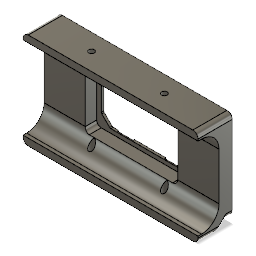
mains_plug_panel-parametric (Autodesk Fusion 360 design; units mm, degrees)
Autodesk Fusion 360 part; units mm, degrees
sketch "Sketch1" plane through (0, 0, 0) normal (1, 0, 0) x (0, 0, -1)
  line L0 (0, 0) -> (0, 51)
  line L1 (0, 51) -> (-20, 51)
  line L2 (-20, 51) -> (-20, 47)
  line L3 (-20, 47) -> (-18, 47)
  line L4 (-18, 47) -> (-8, 47) construction
  line L5 (-8, 47) -> (-8, 37) construction
  arc A0 (-8, 37) -> (-18, 47) centre (-18, 37) ccw
  line L6 (-8, 37) -> (-8, 10)
  line L7 (0, 0) -> (-7, 0)
  line L8 (-7, 0) -> (-11, 0) construction
  line L9 (-11, 0) -> (-11, -4) construction
  line L10 (-7, 0) -> (-11, -4)
  line L11 (-11, -4) -> (-20, -4)
  line L12 (-20, -4) -> (-20, 0)
  line L13 (-20, 0) -> (-18, 0)
  line L14 (-18, 0) -> (-8, 0) construction
  line L15 (-8, 0) -> (-8, 10) construction
  arc A1 (-18, 0) -> (-8, 10) centre (-18, 10) ccw
  line L16 (-8, 10) -> (0, 10) construction
  dimension "d1" = 51
  dimension "d2" = 20
  dimension "d3" = 4
  dimension "d5" = 2
  dimension "d6" = 10
  dimension "d7" = 10
  dimension "d8" = 27
  dimension "d12" = 7
  dimension "d13" = 4
  dimension "d14" = 4
  dimension "d15" = 9
  dimension "d16" = 4
  dimension "d17" = 2
  dimension "d18" = 10
  dimension "d19" = 10
  measures "d1" distance of L0.start
  measures "d2" distance of L0.start
  measures "d5" distance of L0.start
  measures "d12" distance of L0.start
  measures "d16" distance of L0.start
  measures "d17" distance of L0.start
extrude "Extrude1" add sketch "Sketch1" along normal blind 100
sketch "Sketch3" plane through (0, 0, 20) normal (0, 0, 1) x (1, 0, 0)
  line L0 (0, 51) -> (0, 47)
  line L1 (0, 47) -> (100, 47)
  line L2 (100, 47) -> (100, 51)
  line L3 (100, 51) -> (0, 51)
  line L4 (0, -4) -> (100, -4)
  line L5 (50, 51) -> (50, -4) construction
  line L6 (23.6, 39.5815) -> (76.4, 39.5815)
  line L7 (76.4, 39.5815) -> (76.4, 7.4185)
  line L8 (76.4, 7.4185) -> (23.6, 7.4185)
  line L9 (23.6, 7.4185) -> (23.6, 39.5815)
  line L10 (50, 23.5) -> (23.6, 23.5) construction
  line L11 (50, 23.5) -> (76.4, 23.5) construction
  dimension "d22" = 52.8
  dimension "d23" = 32.163
  measures "d23" distance of origin
extrude "Extrude2" cut sketch "Sketch3" against normal blind 18.5 contours L6 L7 L8 L9
fillet "Fillet1" radius 2.6 4 edges at (76.4, 39.5815, 4.9195) (23.6, 39.5815, 4.9195) (23.6, 7.4185, 4.9195) (76.4, 7.4185, 4.9195)
sketch "Sketch4" plane through (0, 0, 20) normal (0, 0, 1) x (1, 0, 0)
  line L0 (0, 51) -> (0, 47)
  line L1 (0, 47) -> (100, 47)
  line L2 (100, 47) -> (100, 51)
  line L3 (100, 51) -> (0, 51)
  line L4 (0, -4) -> (100, -4)
  line L5 (50, 51) -> (50, -4) construction
  line L6 (26.3, 37.25) -> (73.7, 37.25)
  line L7 (73.7, 37.25) -> (73.7, 9.75)
  line L8 (73.7, 9.75) -> (26.3, 9.75)
  line L9 (26.3, 9.75) -> (26.3, 37.25)
  line L10 (50, 23.5) -> (26.3, 23.5) construction
  line L11 (50, 23.5) -> (73.7, 23.5) construction
  dimension "d27" = 47.4
  dimension "d28" = 27.5
  measures "d28" distance of origin
extrude "Extrude3" cut sketch "Sketch4" against normal blind 26 contours L6 L7 L8 L9
chamfer "Chamfer2" distance 5 angle 45 2 edges at (26.3, 9.75, 0.75) (26.3, 37.25, 0.75)
fillet "Fillet3" radius 0.894 6 edges at (31.3, 37.25, 0.75) (26.3, 32.25, 0.75) (26.3, 14.75, 0.75) (31.3, 9.75, 0.75) (73.7, 37.25, 0.75) (73.7, 9.75, 0.75)
sketch "Sketch5" plane through (0, 51, 0) normal (0, 1, 0) x (-1, 0, 0)
  line L0 (0, 0) -> (0, 20)
  line L1 (0, 20) -> (-100, 20)
  line L2 (-100, 20) -> (-100, 0)
  line L3 (-100, 0) -> (0, 0)
  line L4 (-50, 10) -> (-29.1875, 10) construction
  line L5 (-50, 10) -> (-70.8125, 10.025) construction
  circle A0 centre (-70.8125, 10.025) radius 1.6
  circle A1 centre (-29.1875, 10) radius 1.6
  line L6 (-50, 10) -> (-50, 0) construction
  dimension "d35" = 20.8125
  dimension "d36" = 20.8125
  dimension "d37" = 3.2
  dimension "d38" = 3.2
  dimension "d41" = 10
  measures "d37" diameter of A0
  measures "d38" diameter of A1
  measures "d41" distance of L0.start
sketch "Sketch7" plane through (0, 0, 0) normal (0, 0, -1) x (-1, 0, 0)
  line L0 (-73.7, 10.644) -> (-73.7, 36.356)
  arc A0 (-72.806, 37.25) -> (-73.7, 36.356) centre (-72.806, 36.356) ccw
  line L1 (-72.806, 37.25) -> (-31.6703, 37.25)
  arc A1 (-31.0382, 36.9882) -> (-31.6703, 37.25) centre (-31.6703, 36.356) ccw
  line L2 (-31.0382, 36.9882) -> (-26.5618, 32.5118)
  arc A2 (-26.3, 31.8797) -> (-26.5618, 32.5118) centre (-27.194, 31.8797) ccw
  line L3 (-26.3, 31.8797) -> (-26.3, 15.1203)
  arc A3 (-26.5618, 14.4882) -> (-26.3, 15.1203) centre (-27.194, 15.1203) ccw
  line L4 (-26.5618, 14.4882) -> (-31.0382, 10.0118)
  arc A4 (-31.6703, 9.75) -> (-31.0382, 10.0118) centre (-31.6703, 10.644) ccw
  line L5 (-31.6703, 9.75) -> (-72.806, 9.75)
  arc A5 (-73.7, 10.644) -> (-72.806, 9.75) centre (-72.806, 10.644) ccw
  line L6 (0, 0) -> (0, 51)
  line L7 (0, 51) -> (-100, 51)
  line L8 (-100, 51) -> (-100, 0)
  line L9 (-100, 0) -> (0, 0)
  line L10 (-71.7, 38.75) -> (-61.7, 38.75)
  line L11 (-61.7, 38.75) -> (-61.7, 8.25)
  line L12 (-61.7, 8.25) -> (-71.7, 8.25)
  line L13 (-71.7, 8.25) -> (-71.7, 38.75)
  line L14 (-66.7, 38.75) -> (-66.7, 37.25) construction
  line L15 (-66.7, 8.25) -> (-66.7, 9.75) construction
  line L16 (-71.7, 22) -> (-73.7, 22) construction
  line L17 (-43.7, 38.75) -> (-34.7, 38.75)
  line L18 (-34.7, 38.75) -> (-34.7, 8.25)
  line L19 (-34.7, 8.25) -> (-43.7, 8.25)
  line L20 (-43.7, 8.25) -> (-43.7, 38.75)
  line L21 (-73.7, 23.5) -> (-43.7, 23.5) construction
  dimension "d51" = 30.5
  dimension "d52" = 2
  dimension "d53" = 10
  dimension "d54" = 30
  dimension "d55" = 9
  measures "d51" distance of L6.start
  measures "d54" distance of L6.start
extrude "Extrude6" cut sketch "Sketch7" against normal blind 0.75 contours L5 L11 L12 L13 | L1 L10 L11 L13 | L5 L18 L19 L20 | L1 L17 L18 L20
extrude "Extrude4" cut sketch "Sketch5" against normal blind 77 contours A0 | A1
fillet "Fillet4" radius 3 6 edges at (0, 51, 10) (0, -4, 15.5) (100, -4, 15.5) (100, 51, 10) (100, 0, 3.5) (0, 0, 3.5)
chamfer "Chamfer3" distance 0.4 angle 45 8 edges at (50, 51, 0) (0.8787, 50.1213, 0) (0, 25.5, 0) (0.8787, 0.8787, 0) (50, 0, 0) (99.1213, 0.8787, 0) (100, 25.5, 0) (99.1213, 50.1213, 0)
sketch "Sketch6" plane through (0, 51, 0) normal (0, 1, 0) x (-1, 0, 0)
  line L0 (-97, 0.4) -> (-3, 0.4)
  line L1 (-3, 0.4) -> (-3, 20)
  line L2 (-3, 20) -> (-97, 20)
  line L3 (-97, 20) -> (-97, 0.4)
  circle A0 centre (-70.8125, 10.025) radius 1.6
  circle A1 centre (-29.1875, 10) radius 1.6
  circle A2 centre (-29.1875, 10) radius 3
  circle A3 centre (-70.8125, 10.025) radius 3
  dimension "d44" = 6
  dimension "d45" = 6
  measures "d44" diameter of A2
  measures "d45" diameter of A3
extrude "Extrude5" cut sketch "Sketch6" against normal blind 15 from surface at -4 contours A0 | A1 | A2 | A3
chamfer "Chamfer4" distance 0.5 angle 45 4 edges at (66.7, 38.75, 0.75) (39.2, 38.75, 0.75) (39.2, 8.25, 0.75) (66.7, 8.25, 0.75)
equation "d20 = Panel_Length"
equation "d35 = ( 41.625 / 2 ) * 1 mm"
equation "d36 = ( 41.625 / 2 ) * 1 mm"
equation "Panel_Length = 100 mm"
